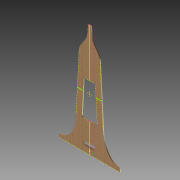
# Autodesk Inventor part: Top Plate
Saved by Autodesk Inventor 2013 SP1 (Build 170176100, 176)
## iProperties
Created: 2013-02-28
Part Number: Top Plate
Material: Wood (Cherry)
Document SubType Name: Modeling
Designer: fixer
Mass: 47.8412 g
Surface Area: 653.113 cm^2
Volume: 95.6825 cm^3
Density: 0.5 g/cm^3
Author: fixer
Autodesk Inventor part; units mm, degrees
ref_plane "YZ Plane" through (0, 0, 0) normal (1, 0, 0) x (0, 1, 0)
ref_plane "XZ Plane" through (0, 0, 0) normal (0, 1, 0) x (-1, 0, 0)
ref_plane "XY Plane" through (0, 0, 0) normal (0, 0, 1) x (1, 0, 0)
derived "Bottom Plate v2.ipt"
sketch "Sketch1_1" plane through (0, 0, 0) normal (0, 0, 1) x (1, 0, 0)
  line L0 (76.2, -12.7) -> (381, -12.7) construction
  line L1 (-76.2, -12.7) -> (-381, -12.7) construction
  line L2 (-76.2, 0) -> (-381, 0) construction
  line L3 (76.2, 0) -> (381, 0) construction
  line L4 (0, -116.2267) -> (0, 608.4603) construction
  line L5 (0, -12.7) -> (-114.3, -12.7)
  line L6 (-114.3, -12.7) -> (-114.3, 0)
  line L7 (0, 406.4) -> (-6.35, 406.4)
  line L8 (-39.0138, 312.42) -> (-50.5988, 93.6374)
  line L9 (39.0138, 312.42) -> (50.5988, 93.6374)
  line L10 (0, 406.4) -> (6.35, 406.4)
  line L11 (0, -12.7) -> (114.3, -12.7)
  line L12 (114.3, -12.7) -> (114.3, 0)
  spline S0 degree 4 poles (-6.35, 406.4) (-6.35, 381.154) (-10.7035, 365.7003) (-9.9482, 354.3709) (-38.2791, 326.2946) (-39.0138, 312.42) knots 0 0 0 0 0 0.492384 1 1 1 1 1
  spline S1 degree 4 poles (6.35, 406.4) (6.35, 381.154) (10.7035, 365.7003) (9.9482, 354.3709) (38.2791, 326.2946) (39.0138, 312.42) knots 0 0 0 0 0 0.492384 1 1 1 1 1
  spline S2 degree 3 poles (-50.5988, 93.6374) (-52.7393, 53.2143) (-67.314, 0) (-114.3, 0) knots 0 0 0 0 1 1 1 1
  spline S3 degree 3 poles (50.5988, 93.6374) (52.7393, 53.2143) (67.314, 0) (114.3, 0) knots 0 0 0 0 1 1 1 1
  line L13 (19.05, 12.7) -> (-19.05, 12.7)
  line L14 (-19.05, 12.7) -> (-19.05, 23.9218)
  line L15 (-19.05, 23.9218) -> (19.05, 23.9218)
  line L16 (19.05, 23.9218) -> (19.05, 12.7)
  line L17 (-19.05, 20.9628) -> (19.05, 20.9628) construction
  line L18 (-12.7, 168.7226) -> (-12.7, 228.9206) construction
  line L19 (12.7, 168.7226) -> (-12.7, 168.7226) construction
  line L20 (12.7, 228.9206) -> (12.7, 168.7226) construction
  line L21 (-12.7, 228.9206) -> (12.7, 228.9206) construction
  line L22 (-47.625, 12.7) -> (47.625, 12.7) construction
  line L23 (0, 96.1517) -> (23.388, 96.1517)
  line L24 (28.4609, 101.5003) -> (22.0411, 222.7364)
  line L25 (16.9683, 227.5478) -> (0, 227.5478)
  line L26 (0, 96.1517) -> (-23.388, 96.1517)
  line L27 (-28.4609, 101.5003) -> (-22.0411, 222.7364)
  line L28 (-16.9683, 227.5478) -> (0, 227.5478)
  arc A0 (-16.9683, 227.5478) -> (-22.0411, 222.7364) centre (-16.9683, 222.4678) ccw
  arc A1 (22.0411, 222.7364) -> (16.9683, 227.5478) centre (16.9683, 222.4678) ccw
  arc A2 (23.388, 96.1517) -> (28.4609, 101.5003) centre (23.388, 101.2317) ccw
  arc A3 (-28.4609, 101.5003) -> (-23.388, 96.1517) centre (-23.388, 101.2317) ccw
  point P0 (0, 0)
  point P1 (-12.9192, 359.3339)
  point P2 (12.9192, 359.3339)
  point P3 (0, 12.7)
  point P4 (28.7441, 96.1517)
  point P5 (21.7864, 227.5478)
  point P6 (-28.7441, 96.1517)
  point P7 (-21.7864, 227.5478)
  dimension "d9" = 5.08
  measures "d9" radius of A0
extrude "Extrusion2" add sketch "Sketch1_1" along normal blind 3.175
sketch "Etching" plane through (-114.3, -12.7, 3.175) normal (0, 0, 1) x (1, 0, 0)
  line L0 (107.95, 419.1) -> (120.65, 419.1) construction
  line L1 (228.6, 0) -> (0, 0) construction
  line L2 (153.3138, 325.12) -> (164.8988, 106.3374) construction
  line L3 (63.7012, 106.3374) -> (75.2862, 325.12) construction
  line L4 (136.3411, 235.4364) -> (142.7609, 114.2003) construction
  line L5 (85.8391, 114.2003) -> (92.2589, 235.4364) construction
  line L6 (97.3317, 240.2478) -> (131.2683, 240.2478) construction
  line L7 (137.688, 108.8517) -> (90.912, 108.8517) construction
  line L8 (114.3, 419.1) -> (114.3, 240.2478)
  line L9 (114.3, 108.8517) -> (114.3, 0)
  line L10 (68.5015, 196.9911) -> (90.2231, 196.9911)
  line L11 (138.3769, 196.9911) -> (160.0985, 196.9911)
  point P0 (114.3, 12.7)
  point P1 (114.3, 196.9911)
  constraints: 8 end point, 4 midpoint, 4 perpendicular, 4 point on line
body "Solid1"
